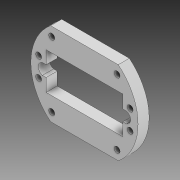
# Autodesk Inventor part: Кронштейн_сервопривод
Saved by Autodesk Inventor 2022 (Build 260153000, 153)
## iProperties
Created: 2025-01-17
Part Number: Кронштейн_сервопривод
Material: Типовые
Document SubType Name: Modeling
Designer: Ivan
Density: 1 g/cm^3
Appearance: По умолчанию
Mass: 8.27311 g
Surface Area: 51.0799 cm^2
Volume: 8.27311 cm^3
Author: Ivan
Title: Кронштейн_сервопривод
Autodesk Inventor part; units mm, degrees
ref_plane "YZ Plane" through (0, 0, 0) normal (1, 0, 0) x (0, 1, 0)
ref_plane "XZ Plane" through (0, 0, 0) normal (0, 1, 0) x (-1, 0, 0)
ref_plane "XY Plane" through (0, 0, 0) normal (0, 0, 1) x (1, 0, 0)
sketch "Эскиз1" plane through (0, 0, 0) normal (0, 0, 1) x (1, 0, 0)
  line L0 (-20.75, 10) -> (20.75, 10)
  line L1 (20.75, 10) -> (20.75, -10)
  line L2 (20.75, -10) -> (-20.75, -10)
  line L3 (-20.75, -10) -> (-20.75, 10)
  line L4 (-20.75, 10) -> (20.75, -10) construction
  line L5 (20.75, 10) -> (-20.75, -10) construction
  circle A0 centre (0, 0) radius 29
  line L6 (0, 0) -> (0, 105.5742) construction
  line L7 (0, 0) -> (104.4464, 0) construction
  circle A1 centre (0, 0) radius 25 construction
  line L8 (0, 0) -> (29.0219, 29.0219) construction
  circle A2 centre (17.6777, 17.6777) radius 1.6
  line L9 (0, 0) -> (-29.0219, 29.0219) construction
  circle A3 centre (-17.6777, 17.6777) radius 1.6
  line L10 (0, 0) -> (-29.0219, -29.0219) construction
  circle A4 centre (-17.6777, -17.6777) radius 1.6
  line L11 (0, 0) -> (29.0219, -29.0219) construction
  circle A5 centre (17.6777, -17.6777) radius 1.6
  circle A6 centre (-24.75, -5.25) radius 1.6
  circle A7 centre (-24.75, 5.25) radius 1.6
  circle A8 centre (24.75, -5.25) radius 1.6
  circle A9 centre (24.75, 5.25) radius 1.6
  line L12 (20.75, 3) -> (22.75, 3)
  line L13 (22.75, 3) -> (22.75, -3)
  line L14 (22.75, -3) -> (20.75, -3)
  line L15 (20.75, -3) -> (20.75, 3)
  line L16 (-20.75, 3) -> (-22.75, 3)
  line L17 (-22.75, 3) -> (-22.75, -3)
  line L18 (-22.75, -3) -> (-20.75, -3)
  line L19 (-20.75, -3) -> (-20.75, 3)
  line L20 (-18.2962, -22.5) -> (18.2962, -22.5)
  line L21 (-18.2962, 22.5) -> (18.2962, 22.5)
  arc A10 (22.75, -3) -> (22.75, 3) centre (21.875, 0) ccw
  arc A11 (-22.75, 3) -> (-22.75, -3) centre (-21.875, 0) ccw
  point P0 (-20.75, -3)
  point P1 (-20.75, 3)
  dimension "d18" = 50
  dimension "d0" = 41.5
  dimension "d1" = 20
  dimension "d8" = 58
  dimension "d17" = 45
  dimension "d19" = 3.2
  dimension "d22" = 360
  dimension "d24" = 3.2
  dimension "d25" = 4.75
  dimension "d26" = 4
  dimension "d29" = 4.75
  dimension "d31" = 2
  dimension "d32" = 6
  dimension "d33" = 2
  dimension "d34" = 45
  constraints: 44 end point, 11 centre point, 8 coincident, 8 point on circle, 7 symmetric about line, 5 horizontal, 4 parallel, 4 point on line, 3 perpendicular, 2 midpoint, 1 equal radius, 1 vertical alignment, 31 other
  measures "d0" distance of L1.end L2.end
  measures "d1" distance of L0.end L1.end
  measures "d8" diameter of A0
  measures "d17" angle of L8 L7
  measures "d19" diameter of A2
  measures "d24" diameter of A6
  measures "d25" distance from line of L2 A6.centre
  measures "d26" distance from line of L3 A6.centre
  measures "d29" distance from line of L0 A7.centre
  measures "d31" distance of L13.end L14.end
  measures "d32" distance of L12.end L13.end
  measures "d33" distance between parallel lines of L1 L13
  measures "d34" distance between parallel lines of L21 L20
extrude "Выдавливание1" add sketch "Эскиз1" along normal mid plane 6 contours A0 L20 L21
